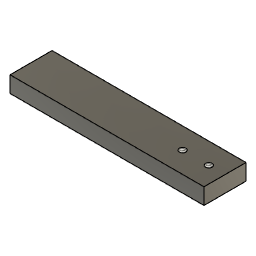
cuboid (Autodesk Fusion 360 design; units mm, degrees)
Autodesk Fusion 360 part; units mm, degrees
sketch "草图1" plane through (0, 0, 0) normal (0, 0, 1) x (1, 0, 0)
  line L0 (30, -6.5) -> (-30, -6.5)
  line L1 (-30, -6.5) -> (-30, 6.5)
  line L2 (-30, 6.5) -> (30, 6.5)
  line L3 (30, 6.5) -> (30, -6.5)
  line L4 (30, -6.5) -> (-30, 6.5) construction
  line L5 (-30, -6.5) -> (30, 6.5) construction
  dimension "d1" = 60
  dimension "d2" = 13
  constraint horizontal L0
  constraint perpendicular L0 L1
  constraint parallel L0 L2
  constraint parallel L1 L3
  constraint coincident L4 origin
  constraint coincident L5 origin
  measures "d1" distance of L1.end L2.end
  measures "d2" distance of L0.end L1.end
extrude "拉伸1" add sketch "草图1" along normal blind 5
hole "孔1" at (0, 0, 5) direction (0, 0, -1) diameter 2.076 depth 10 tip angle 180
thread "螺纹1" "ISO Metric profile 2.5 M2.5x0.45 6H" thread offset 0 thread depth 9
move_face "MoveFace1" to x (1, 0, 0) y (0, 1, 0) z (0, 0, 1) at (25, 0, 0) 1 faces at (0.0517, -1.0367, 3.3333)
hole "孔2" at (-0.1089, 0, 5) direction (0, 0, -1) diameter 2.076 depth 10 tip angle 180
thread "螺纹2" "ISO Metric profile 2.5 M2.5x0.45 6H" thread offset 0 thread depth 9
move_face "MoveFace2" to x (1, 0, 0) y (0, 1, 0) z (0, 0, 1) at (17, 0, 0) 1 faces at (-0.0572, -1.0367, 3.3333)
